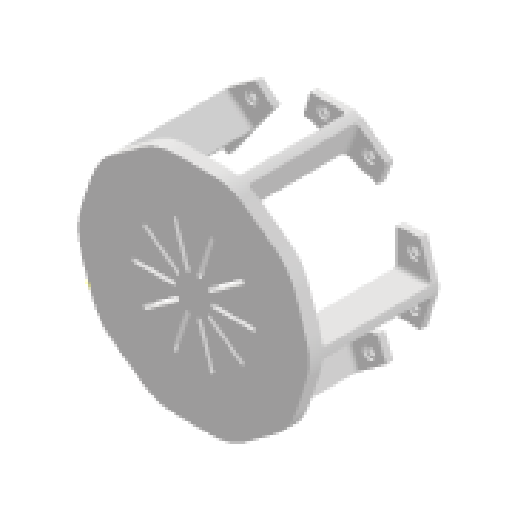
# Autodesk Inventor part: lidarCageTop
Saved by Autodesk Inventor 2025 (Build 290162000, 162)
## iProperties
Created: 2024-12-09
Part Number: lidarCageTop
Material: Generic
Document SubType Name: Modeling
Designer: derm
Density: 1 g/cm^3
Appearance: Default
Author: derm
Autodesk Inventor part; units mm, degrees
ref_plane "YZ Plane" through (0, 0, 0) normal (1, 0, 0) x (0, 1, 0)
ref_plane "XZ Plane" through (0, 0, 0) normal (0, 1, 0) x (-1, 0, 0)
ref_plane "XY Plane" through (0, 0, 0) normal (0, 0, 1) x (1, 0, 0)
sketch "Sketch1" plane through (0, 0, 0) normal (0, 0, 1) x (1, 0, 0)
  line L0 (-28.7185, 88.3865) -> (-75.186, 54.6258) projected
  line L1 (-75.186, 54.6258) -> (-92.935, 0) projected
  line L2 (-92.935, 0) -> (-75.186, -54.6258) projected
  line L3 (-75.186, -54.6258) -> (-28.7185, -88.3865) projected
  line L4 (-28.7185, -88.3865) -> (28.7185, -88.3865) projected
  line L5 (28.7185, -88.3865) -> (75.186, -54.6258) projected
  line L6 (75.186, -54.6258) -> (92.935, 0) projected
  line L7 (92.935, 0) -> (75.186, 54.6258) projected
  line L8 (75.186, 54.6258) -> (28.7185, 88.3865) projected
  line L9 (28.7185, 88.3865) -> (-28.7185, 88.3865) projected
  circle A0 centre (0, 0) radius 52 projected
  line L10 (68.094, 49.4732) -> (84.1688, 0)
  line L11 (84.1688, 0) -> (68.094, -49.4732)
  line L12 (68.094, -49.4732) -> (26.0096, -80.0493)
  line L13 (26.0096, -80.0493) -> (-26.0096, -80.0493)
  line L14 (-26.0096, -80.0493) -> (-68.094, -49.4732)
  line L15 (-68.094, -49.4732) -> (-84.1688, 0)
  line L16 (-84.1688, 0) -> (-68.094, 49.4732)
  line L17 (-68.094, 49.4732) -> (-26.0096, 80.0493)
  line L18 (-26.0096, 80.0493) -> (26.0096, 80.0493)
  line L19 (26.0096, 80.0493) -> (68.094, 49.4732)
  line L20 (58.9142, 0) -> (47.6626, 34.6289)
  line L21 (47.6626, 34.6289) -> (18.2055, 56.0308)
  line L22 (18.2055, 56.0308) -> (-18.2055, 56.0308)
  line L23 (-18.2055, 56.0308) -> (-47.6626, 34.6289)
  line L24 (-47.6626, 34.6289) -> (-58.9142, 0)
  line L25 (-58.9142, 0) -> (-47.6626, -34.6289)
  line L26 (-47.6626, -34.6289) -> (-18.2055, -56.0308)
  line L27 (-18.2055, -56.0308) -> (18.2055, -56.0308)
  line L28 (18.2055, -56.0308) -> (47.6626, -34.6289)
  line L29 (47.6626, -34.6289) -> (58.9142, 0)
  circle A1 centre (0, 0) radius 3
  line L30 (0, 0) -> (82.9915, -3.6235)
  line L31 (0, 0) -> (41.045, 0)
  line L32 (0, 0) -> (82.9915, 3.6235)
  line L33 (58.0901, 2.5363) -> (58.0901, -2.5363)
  point P0 (0, 0)
  dimension "d0" = 6
  dimension "d1" = 2.5
  dimension "d2" = 2.5
  constraints: 48 end point, 6 point on line, 1 centre point, 1 coincident, 1 horizontal, 18 other
  measures "d0" diameter of A1
  measures "d1" angle of L31 L32
  measures "d2" angle of L30 L31
extrude "Extrusion1" add sketch "Sketch1" along normal blind 83 contours L32 L10 L11 L30 L29 L20 | L20 L29 L33
ref_plane "Work Plane1" through (-69.2713, -45.8497, 83) normal (0, 0, 1) x (0.8338858, 0.551937, 0)
sketch "Sketch2" plane through (-69.2713, -45.8497, 83) normal (0, 0, 1) x (0.8338858, 0.551937, 0)
  line L0 (105.8546, 82.1566) -> (53.2128, 79.8582) projected
  line L1 (53.2128, 79.8582) -> (11.9756, 47.0567) projected
  line L2 (11.9756, 47.0567) -> (-2.1057, -3.7189) projected
  line L3 (-2.1057, -3.7189) -> (16.3474, -53.074) projected
  line L4 (16.3474, -53.074) -> (60.2865, -82.1566) projected
  line L5 (60.2865, -82.1566) -> (112.9283, -79.8582) projected
  line L6 (112.9283, -79.8582) -> (154.1655, -47.0567) projected
  line L7 (154.1655, -47.0567) -> (168.2468, 3.7189) projected
  line L8 (168.2468, 3.7189) -> (149.7937, 53.074) projected
  line L9 (149.7937, 53.074) -> (105.8546, 82.1566) projected
  circle A0 centre (83.0705, 0) radius 52 projected
  point P0 (83.0705, 0)
extrude "Extrusion2" add sketch "Sketch2" along normal blind 10 contours L9 L8 L7 L6 L5 L4 L3 L2 L1 L0 | A0
sketch "Sketch3" plane through (-69.2713, -45.8497, 83) normal (0, 0, -1) x (-0.8338858, -0.551937, 0)
  circle A0 centre (-83.0705, 0) radius 52 projected
  point P0 (-83.0705, 0)
extrude "Extrusion3" cut sketch "Sketch3" against normal blind 2
fillet "Fillet1" radius 3 2 edges at (70.5408, 3.0799, 83) (70.5408, -3.0799, 83)
sketch "Sketch4" plane through (0, 0, 0) normal (0, 0, -1) x (-1, 0, 0)
  line L0 (-82.9915, 3.6235) -> (-58.0901, 2.5363) projected
  line L1 (-84.1688, 0) -> (-82.9915, 3.6235) projected
  line L2 (-82.9915, -3.6235) -> (-84.1688, 0) projected
  line L3 (-58.0901, -2.5363) -> (-82.9915, -3.6235) projected
  line L4 (-58.0901, 2.5363) -> (-58.0901, -2.5363) projected
  line L5 (-84.1688, 0) -> (-74.8462, -28.6921)
  line L6 (-84.1688, 0) -> (-58.0901, 80.2619)
  line L7 (-58.0901, 5.5391) -> (-58.0901, -5.5391) projected
  line L8 (-58.0901, -2.5363) -> (-58.0901, -5.5391)
  line L9 (-58.0901, -5.5391) -> (-82.0294, -6.5843)
  line L10 (-82.0294, -6.5843) -> (-58.0901, -5.5391) projected
  line L11 (-82.0294, 6.5843) -> (-58.0901, 5.5391)
  line L12 (-58.0901, -5.5391) -> (-58.0901, 5.5391)
  line L13 (-58.0901, -5.5391) -> (-58.0901, -12.5556)
  line L14 (-74.8462, -28.6921) -> (-58.0901, -27.9605)
  line L15 (-74.8462, 28.6921) -> (-57.9573, 27.9547)
  line L16 (-58.0901, -12.5556) -> (-58.0901, -27.9605)
  line L17 (-58.0901, 5.5391) -> (-57.9573, 27.9547)
  line L18 (-70.0598, -28.4831) -> (-70.0598, -6.0617) construction
  line L19 (-70.0598, 6.0617) -> (-70.0598, 28.4831) construction
  circle A0 centre (-70.0598, -17.2724) radius 2.75
  circle A1 centre (-70.0598, 17.2724) radius 2.75
  point P0 (0, 0)
  point P1 (-80.858, -13.5399)
  point P2 (-70.5408, 3.0799)
  dimension "d15" = 25.4
  dimension "d16" = 25.4
  dimension "d21" = 5.5
  dimension "d22" = 5.5
  constraints: 26 end point, 9 point on line, 5 midpoint, 3 parallel, 2 centre point, 2 collinear, 1 vertical, 2 other
  measures "d15" distance between parallel lines of L14 L3
  measures "d16" distance from line of L15 point (-70.541, 3.08)
  measures "d21" diameter of A0
  measures "d22" diameter of A1
extrude "Extrusion4" add sketch "Sketch4" against normal blind 5
fillet "Fillet2" radius 3 2 edges at (70.5408, 3.0799, 5) (70.5408, -3.0799, 5)
pattern_circular "Circular Pattern2" count 5 over 360 about axis through (0, 0, 83) along (0, 0, 1) of "Extrusion1", "Fillet1", "Extrusion4", "Fillet2"
sketch "Sketch5" plane through (-69.2713, -45.8497, 93) normal (0, 0, 1) x (0.8338858, 0.551937, 0)
  circle A0 centre (83.0705, 0) radius 52 projected
  line L0 (125.8114, 1.8661) -> (97.3202, 0.6222) construction
  line L1 (125.7426, 3.441) -> (97.2514, 2.1971)
  line L2 (97.3889, -0.9528) -> (125.8801, 0.2912)
  arc A1 (125.8801, 0.2912) -> (125.7426, 3.441) centre (125.8114, 1.8661) ccw
  arc A2 (97.2514, 2.1971) -> (97.3889, -0.9528) centre (97.3202, 0.6222) ccw
  line L3 (154.1655, -47.0567) -> (168.2468, 3.7189) projected
  line L4 (168.2468, 3.7189) -> (83.0705, 0) construction
  point P0 (83.0705, 0)
  point P1 (111.5658, 1.2441)
  constraints: 10 end point, 4 point on circle, 4 tangent, 2 centre point, 1 collinear, 1 midpoint, 1 parallel, 1 point on line
extrude "Extrusion5" cut sketch "Sketch5" against normal up to surface (10 mm away) contours A1 L2 A2 L1
pattern_circular "Circular Pattern3" count 10 over 360 about axis through (0, 0, -10) along (0, 0, 1) of "Extrusion5"
sketch "Sketch6" plane through (-70.2334, 42.8889, 5) normal (0, 0, 1) x (0.8338858, -0.551937, 0)
  circle A0 centre (11.492, -11.2) radius 2.75 projected
  circle A1 centre (12.9989, 23.3119) radius 2.75 projected
  circle A2 centre (12.9989, 23.3119) radius 4.5
  circle A3 centre (11.492, -11.2) radius 4.5
  point P0 (82.2386, 3)
  dimension "d31" = 9
  dimension "d32" = 9
  constraints: 2 centre point, 2 coincident
  measures "d31" diameter of A2
  measures "d32" diameter of A3
extrude "Extrusion6" cut sketch "Sketch6" against normal blind 2
pattern_circular "Circular Pattern4" count 5 over 360 about axis through (0, 0, 83) along (0, 0, 1) of "Extrusion6"
fillet "Fillet3" radius 40 10 edges at (26.346, -81.0846, 88) (68.9747, -50.113, 88) (85.2574, 0, 88) (68.9747, 50.113, 88) (26.346, 81.0846, 88) (-26.346, 81.0846, 88) (-68.9747, 50.113, 88) (-85.2574, 0, 88) (-68.9747, -50.113, 88) (-26.346, -81.0846, 88)
body "Solid1"
